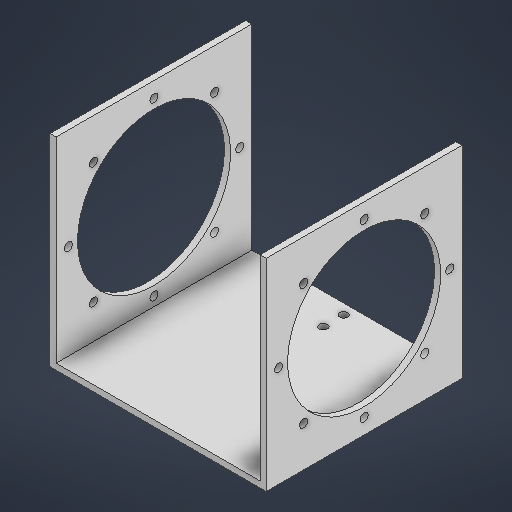
# Autodesk Inventor part: shoulder
Saved by Autodesk Inventor 2026 (Build 300175000, 175)
## iProperties
Created: 2025-07-17
Part Number: shoulder
Material: Generic
Document SubType Name: Modeling
Designer: User
Density: 1 g/cm^3
Appearance: Default
Author: User
Autodesk Inventor part; units mm, degrees
ref_plane "YZ Plane" through (0, 0, 0) normal (1, 0, 0) x (0, 1, 0)
ref_plane "XZ Plane" through (0, 0, 0) normal (0, 1, 0) x (-1, 0, 0)
ref_plane "XY Plane" through (0, 0, 0) normal (0, 0, 1) x (1, 0, 0)
sketch "Sketch2" plane through (0, 0, 0) normal (0, 1, 0) x (-1, 0, 0)
  line L0 (53, 48) -> (-53, 48)
  line L1 (-53, 48) -> (-53, -48)
  line L2 (-53, -48) -> (53, -48)
  line L3 (53, -48) -> (53, 48)
  line L4 (53, 48) -> (-53, -48) construction
  line L5 (-53, 48) -> (53, -48) construction
  point P0 (0, 0)
  dimension "d20" = 106
  dimension "d21" = 96
  constraints: 12 end point, 2 midpoint, 2 parallel, 1 horizontal, 1 perpendicular
  measures "d20" distance of L2.end L1.end
  measures "d21" distance of L1.end L0.end
extrude "Extrusion1" add sketch "Sketch2" along normal blind 3
sketch "Sketch4" plane through (0, 3, 0) normal (0, 1, 0) x (1, 0, 0)
  line L0 (53, -48) -> (53, 48) projected
  line L1 (-53, -48) -> (53, -48) projected
  line L2 (53, 48) -> (50, 48)
  line L3 (50, 48) -> (50, -48)
  line L4 (50, -48) -> (53, -48)
  line L5 (53, -48) -> (53, 48)
  line L6 (53, 48) -> (-53, 48) projected
  line L7 (-53, 48) -> (-50, 48)
  line L8 (-50, 48) -> (-50, -48)
  line L9 (-50, -48) -> (-53, -48)
  line L10 (-53, -48) -> (-53, 48)
  point P0 (0, 0)
  dimension "d22" = 3
  dimension "d45" = 3
  constraints: 16 end point, 4 parallel, 2 horizontal, 2 perpendicular, 2 point on line
  measures "d22" distance of L4.end L3.end
  measures "d45" distance of L8.end L9.end
extrude "Extrusion3" add sketch "Sketch4" along normal blind 96 contours L1 L3 L2 L0 | L1 L10 L6 L8
sketch "Sketch5" plane through (53, 0, 48) normal (1, 0, 0) x (0, 0, -1)
  line L0 (48, 99) -> (48, 0) construction
  line L1 (0, 99) -> (96, 99) projected
  circle A0 centre (48, 49.5) radius 37.5
  dimension "d27" = 75
  constraints: 2 end point, 1 centre point, 1 midpoint, 1 vertical
  measures "d27" diameter of A0
extrude "Extrusion4" cut sketch "Sketch5" against normal blind 164.2625
sketch "Sketch6" plane through (53, 0, 48) normal (1, 0, 0) x (0, 0, -1)
  circle A0 centre (48, 49.5) radius 37.5 projected
  circle A1 centre (48, 49.5) radius 42 construction
  circle A2 centre (90, 49.5) radius 2
  circle A3 centre (48, 49.5) radius 42 construction
  circle A4 centre (77.6985, 79.1985) radius 2
  circle A5 centre (48, 49.5) radius 42 construction
  circle A6 centre (48, 91.5) radius 2
  circle A7 centre (48, 49.5) radius 42 construction
  circle A8 centre (18.3015, 79.1985) radius 2
  circle A9 centre (48, 49.5) radius 42 construction
  circle A10 centre (6, 49.5) radius 2
  circle A11 centre (48, 49.5) radius 42 construction
  circle A12 centre (18.3015, 19.8015) radius 2
  circle A13 centre (48, 49.5) radius 42 construction
  circle A14 centre (48, 7.5) radius 2
  circle A15 centre (48, 49.5) radius 42 construction
  circle A16 centre (77.6985, 19.8015) radius 2
  point P0 (48, 0)
  dimension "d30" = 84
  dimension "d31" = 4
  dimension "d34" = 360
  constraints: 8 centre point, 3 coincident, 2 horizontal alignment, 2 vertical alignment, 51 other
  measures "d31" diameter of A2
extrude "Extrusion5" cut sketch "Sketch6" against normal blind 164.2625 contours A2 | A4 | A6 | A8 | A10 | A12 | A14 | A16
sketch "Sketch7" plane through (0, 0, 0) normal (0, -1, 0) x (1, 0, 0)
  line L0 (53, -48) -> (-53, -48) projected
  line L1 (0, -48) -> (0, -43) construction
  line L2 (0, -43) -> (0, -33) construction
  circle A0 centre (0, -43) radius 2
  circle A1 centre (0, -33) radius 2
  point P0 (0, 0)
  dimension "d38" = 5
  dimension "d39" = 10
  dimension "d40" = 4
  dimension "d41" = 4
  constraints: 4 end point, 2 centre point, 2 coincident, 1 midpoint, 1 point on line, 1 vertical
  measures "d38" distance of L1.start L1.end
  measures "d39" distance of L1.end L2.end
  measures "d40" diameter of A0
  measures "d41" diameter of A1
extrude "Extrusion6" cut sketch "Sketch7" against normal blind 4
body "Solid1"
